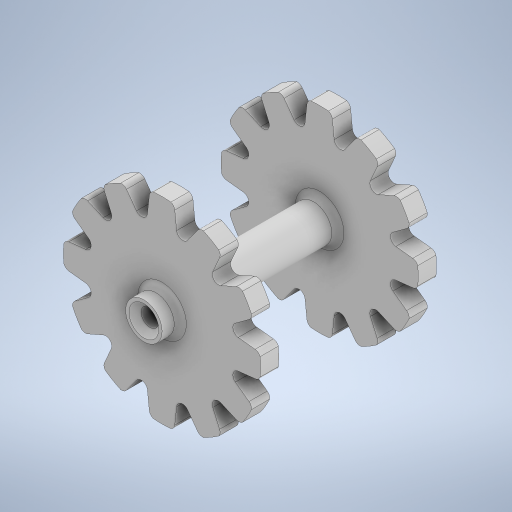
# Autodesk Inventor part: zebatka v12
Saved by Autodesk Inventor 2024 (Build 280153000, 153)
## iProperties
Created: 2025-03-28
Part Number: zebatka v12
Material: Ogólny
Document SubType Name: Modeling
Designer: Victoria
Density: 1 g/cm^3
Appearance: Domyślna
Author: Victoria
Autodesk Inventor part; units mm, degrees
ref_plane "YZ Plane" through (0, 0, 0) normal (1, 0, 0) x (0, 1, 0)
ref_plane "XZ Plane" through (0, 0, 0) normal (0, 1, 0) x (-1, 0, 0)
ref_plane "XY Plane" through (0, 0, 0) normal (0, 0, 1) x (1, 0, 0)
sketch "Szkic1" plane through (0, 0, 0) normal (0, 0, 1) x (1, 0, 0)
  circle A0 centre (0, 0) radius 16.25
  line L0 (0, 16.25) -> (-1.105, 16.25)
  line L1 (0, 16.25) -> (1.105, 16.25)
  line L2 (2.5, 11.75) -> (2.0988, 15.3604)
  line L3 (-2.5, 11.75) -> (-2.0988, 15.3604)
  arc A1 (-1.105, 16.25) -> (-2.0988, 15.3604) centre (-1.105, 15.25) ccw
  arc A2 (2.0988, 15.3604) -> (1.105, 16.25) centre (1.105, 15.25) ccw
  line L4 (3.7099, 11.4258) -> (5.8626, 14.3519)
  arc A3 (7.1681, 14.6254) -> (5.8626, 14.3519) centre (6.6681, 13.7594) ccw
  line L5 (8.125, 14.0729) -> (7.1681, 14.6254)
  line L6 (8.125, 14.0729) -> (9.0819, 13.5204)
  arc A4 (9.4979, 12.2531) -> (9.0819, 13.5204) centre (8.5819, 12.6544) ccw
  line L7 (8.0401, 8.9258) -> (9.4979, 12.2531)
  line L8 (8.9258, 8.0401) -> (12.2531, 9.4979)
  arc A5 (13.5204, 9.0819) -> (12.2531, 9.4979) centre (12.6544, 8.5819) ccw
  line L9 (14.0729, 8.125) -> (13.5204, 9.0819)
  line L10 (14.0729, 8.125) -> (14.6254, 7.1681)
  arc A6 (14.3519, 5.8626) -> (14.6254, 7.1681) centre (13.7594, 6.6681) ccw
  line L11 (11.4258, 3.7099) -> (14.3519, 5.8626)
  line L12 (11.75, 2.5) -> (15.3604, 2.0988)
  arc A7 (16.25, 1.105) -> (15.3604, 2.0988) centre (15.25, 1.105) ccw
  line L13 (16.25, 0) -> (16.25, 1.105)
  line L14 (16.25, 0) -> (16.25, -1.105)
  arc A8 (15.3604, -2.0988) -> (16.25, -1.105) centre (15.25, -1.105) ccw
  line L15 (11.75, -2.5) -> (15.3604, -2.0988)
  line L16 (11.4258, -3.7099) -> (14.3519, -5.8626)
  arc A9 (14.6254, -7.1681) -> (14.3519, -5.8626) centre (13.7594, -6.6681) ccw
  line L17 (14.0729, -8.125) -> (14.6254, -7.1681)
  line L18 (14.0729, -8.125) -> (13.5204, -9.0819)
  arc A10 (12.2531, -9.4979) -> (13.5204, -9.0819) centre (12.6544, -8.5819) ccw
  line L19 (8.9258, -8.0401) -> (12.2531, -9.4979)
  line L20 (8.0401, -8.9258) -> (9.4979, -12.2531)
  arc A11 (9.0819, -13.5204) -> (9.4979, -12.2531) centre (8.5819, -12.6544) ccw
  line L21 (8.125, -14.0729) -> (9.0819, -13.5204)
  line L22 (8.125, -14.0729) -> (7.1681, -14.6254)
  arc A12 (5.8626, -14.3519) -> (7.1681, -14.6254) centre (6.6681, -13.7594) ccw
  line L23 (3.7099, -11.4258) -> (5.8626, -14.3519)
  line L24 (2.5, -11.75) -> (2.0988, -15.3604)
  arc A13 (1.105, -16.25) -> (2.0988, -15.3604) centre (1.105, -15.25) ccw
  line L25 (0, -16.25) -> (1.105, -16.25)
  line L26 (0, -16.25) -> (-1.105, -16.25)
  arc A14 (-2.0988, -15.3604) -> (-1.105, -16.25) centre (-1.105, -15.25) ccw
  line L27 (-2.5, -11.75) -> (-2.0988, -15.3604)
  line L28 (-3.7099, -11.4258) -> (-5.8626, -14.3519)
  arc A15 (-7.1681, -14.6254) -> (-5.8626, -14.3519) centre (-6.6681, -13.7594) ccw
  line L29 (-8.125, -14.0729) -> (-7.1681, -14.6254)
  line L30 (-8.125, -14.0729) -> (-9.0819, -13.5204)
  arc A16 (-9.4979, -12.2531) -> (-9.0819, -13.5204) centre (-8.5819, -12.6544) ccw
  line L31 (-8.0401, -8.9258) -> (-9.4979, -12.2531)
  line L32 (-8.9258, -8.0401) -> (-12.2531, -9.4979)
  arc A17 (-13.5204, -9.0819) -> (-12.2531, -9.4979) centre (-12.6544, -8.5819) ccw
  line L33 (-14.0729, -8.125) -> (-13.5204, -9.0819)
  line L34 (-14.0729, -8.125) -> (-14.6254, -7.1681)
  arc A18 (-14.3519, -5.8626) -> (-14.6254, -7.1681) centre (-13.7594, -6.6681) ccw
  line L35 (-11.4258, -3.7099) -> (-14.3519, -5.8626)
  line L36 (-11.75, -2.5) -> (-15.3604, -2.0988)
  arc A19 (-16.25, -1.105) -> (-15.3604, -2.0988) centre (-15.25, -1.105) ccw
  line L37 (-16.25, 0) -> (-16.25, -1.105)
  line L38 (-16.25, 0) -> (-16.25, 1.105)
  arc A20 (-15.3604, 2.0988) -> (-16.25, 1.105) centre (-15.25, 1.105) ccw
  line L39 (-11.75, 2.5) -> (-15.3604, 2.0988)
  line L40 (-11.4258, 3.7099) -> (-14.3519, 5.8626)
  arc A21 (-14.6254, 7.1681) -> (-14.3519, 5.8626) centre (-13.7594, 6.6681) ccw
  line L41 (-14.0729, 8.125) -> (-14.6254, 7.1681)
  line L42 (-14.0729, 8.125) -> (-13.5204, 9.0819)
  arc A22 (-12.2531, 9.4979) -> (-13.5204, 9.0819) centre (-12.6544, 8.5819) ccw
  line L43 (-8.9258, 8.0401) -> (-12.2531, 9.4979)
  line L44 (-8.0401, 8.9258) -> (-9.4979, 12.2531)
  arc A23 (-9.0819, 13.5204) -> (-9.4979, 12.2531) centre (-8.5819, 12.6544) ccw
  line L45 (-8.125, 14.0729) -> (-9.0819, 13.5204)
  line L46 (-8.125, 14.0729) -> (-7.1681, 14.6254)
  arc A24 (-5.8626, 14.3519) -> (-7.1681, 14.6254) centre (-6.6681, 13.7594) ccw
  line L47 (-3.7099, 11.4258) -> (-5.8626, 14.3519)
  circle A25 centre (0, 0) radius 12.013
  circle A26 centre (0, 0) radius 1.45
  point P0 (-2, 16.25)
  point P1 (2, 16.25)
  point P2 (6.3929, 15.0729)
  point P3 (9.8571, 13.0729)
  point P4 (13.0729, 9.8571)
  point P5 (15.0729, 6.3929)
  point P6 (16.25, 2)
  point P7 (16.25, -2)
  point P8 (15.0729, -6.3929)
  point P9 (13.0729, -9.8571)
  point P10 (9.8571, -13.0729)
  point P11 (6.3929, -15.0729)
  point P12 (2, -16.25)
  point P13 (-2, -16.25)
  point P14 (-6.3929, -15.0729)
  point P15 (-9.8571, -13.0729)
  point P16 (-13.0729, -9.8571)
  point P17 (-15.0729, -6.3929)
  point P18 (-16.25, -2)
  point P19 (-16.25, 2)
  point P20 (-15.0729, 6.3929)
  point P21 (-13.0729, 9.8571)
  point P22 (-9.8571, 13.0729)
  point P23 (-6.3929, 15.0729)
  point P24 (14.7468, 6.826)
  point P25 (13.2849, 9.3581)
  point P26 (9.3581, 13.2849)
  point P27 (6.826, 14.7468)
  point P28 (1.462, 16.1841)
  point P29 (-1.462, 16.1841)
  point P30 (-6.826, 14.7468)
  point P31 (-9.3581, 13.2849)
  point P32 (-13.2849, 9.3581)
  point P33 (-14.7468, 6.826)
  point P34 (-16.1841, 1.462)
  point P35 (-16.1841, -1.462)
  point P36 (-14.7468, -6.826)
  point P37 (-13.2849, -9.3581)
  point P38 (-9.3581, -13.2849)
  point P39 (-6.826, -14.7468)
  point P40 (-1.462, -16.1841)
  point P41 (1.462, -16.1841)
  point P42 (6.826, -14.7468)
  point P43 (9.3581, -13.2849)
  point P44 (13.2849, -9.3581)
  point P45 (14.7468, -6.826)
  point P46 (16.1841, -1.462)
  point P47 (16.1841, 1.462)
  dimension "d0" = 32.5
  dimension "d2" = 2
  dimension "d3" = 2
  dimension "d6" = 1
  dimension "d9" = 360
  dimension "d11" = 2.9
  constraints: 96 end point, 60 point on line, 48 point on circle, 25 centre point, 4 coincident, 4 tangent, 2 horizontal, 1 equal radius, 221 other
  measures "d2" distance of L0.start point (-2, 16.25)
  measures "d3" distance of L0.start point (2, 16.25)
  measures "d6" radius of A1
  measures "d11" diameter of A26
extrude "Wyciągnięcie proste1" add sketch "Szkic1" along normal blind 3 contours A0 A8 L15 A25 L12 A7 | A6 L11 A25 L8 A5 A0 | A0 A10 L19 A25 L16 A9 | A25 | A4 L7 A25 L4 A3 A0 | A0 A12 L23 A25 L20 A11 | A2 L2 A25 L3 A1 A0 | A0 A14 L27 A25 L24 A13 | A25 L44 A23 A0 A24 L47 | L28 A15 A0 A16 L31 A25 | A25 L40 A21 A0 A22 L43 | L32 A17 A0 A18 L35 A25 | A25 L36 A19 A0 A20 L39
sketch "Szkic2" plane through (0, 0, 3) normal (0, 0, 1) x (1, 0, 0)
  circle A0 centre (0, 0) radius 3
  line L0 (11.4258, 3.7099) -> (14.3519, 5.8626) projected
  arc A1 (14.3519, 5.8626) -> (14.7468, 6.826) centre (13.7594, 6.6681) ccw projected
  arc A2 (14.7468, 6.826) -> (13.2849, 9.3581) centre (0, 0) ccw projected
  arc A3 (13.2849, 9.3581) -> (12.2531, 9.4979) centre (12.6544, 8.5819) ccw projected
  line L1 (12.2531, 9.4979) -> (8.9258, 8.0401) projected
  arc A4 (8.9258, 8.0401) -> (8.0401, 8.9258) centre (0, 0) ccw projected
  line L2 (8.0401, 8.9258) -> (9.4979, 12.2531) projected
  arc A5 (9.4979, 12.2531) -> (9.3581, 13.2849) centre (8.5819, 12.6544) ccw projected
  arc A6 (9.3581, 13.2849) -> (6.826, 14.7468) centre (0, 0) ccw projected
  arc A7 (6.826, 14.7468) -> (5.8626, 14.3519) centre (6.6681, 13.7594) ccw projected
  line L3 (5.8626, 14.3519) -> (3.7099, 11.4258) projected
  arc A8 (3.7099, 11.4258) -> (2.5, 11.75) centre (0, 0) ccw projected
  line L4 (2.5, 11.75) -> (2.0988, 15.3604) projected
  arc A9 (2.0988, 15.3604) -> (1.462, 16.1841) centre (1.105, 15.25) ccw projected
  arc A10 (1.462, 16.1841) -> (-1.462, 16.1841) centre (0, 0) ccw projected
  arc A11 (-1.462, 16.1841) -> (-2.0988, 15.3604) centre (-1.105, 15.25) ccw projected
  line L5 (-2.0988, 15.3604) -> (-2.5, 11.75) projected
  arc A12 (-2.5, 11.75) -> (-3.7099, 11.4258) centre (0, 0) ccw projected
  line L6 (-3.7099, 11.4258) -> (-5.8626, 14.3519) projected
  arc A13 (-5.8626, 14.3519) -> (-6.826, 14.7468) centre (-6.6681, 13.7594) ccw projected
  arc A14 (-6.826, 14.7468) -> (-9.3581, 13.2849) centre (0, 0) ccw projected
  arc A15 (-9.3581, 13.2849) -> (-9.4979, 12.2531) centre (-8.5819, 12.6544) ccw projected
  line L7 (-9.4979, 12.2531) -> (-8.0401, 8.9258) projected
  arc A16 (-8.0401, 8.9258) -> (-8.9258, 8.0401) centre (0, 0) ccw projected
  line L8 (-8.9258, 8.0401) -> (-12.2531, 9.4979) projected
  arc A17 (-12.2531, 9.4979) -> (-13.2849, 9.3581) centre (-12.6544, 8.5819) ccw projected
  arc A18 (-13.2849, 9.3581) -> (-14.7468, 6.826) centre (0, 0) ccw projected
  arc A19 (-14.7468, 6.826) -> (-14.3519, 5.8626) centre (-13.7594, 6.6681) ccw projected
  line L9 (-14.3519, 5.8626) -> (-11.4258, 3.7099) projected
  arc A20 (-11.4258, 3.7099) -> (-11.75, 2.5) centre (0, 0) ccw projected
  line L10 (-11.75, 2.5) -> (-15.3604, 2.0988) projected
  arc A21 (-15.3604, 2.0988) -> (-16.1841, 1.462) centre (-15.25, 1.105) ccw projected
  arc A22 (-16.1841, 1.462) -> (-16.1841, -1.462) centre (0, 0) ccw projected
  arc A23 (-16.1841, -1.462) -> (-15.3604, -2.0988) centre (-15.25, -1.105) ccw projected
  line L11 (-15.3604, -2.0988) -> (-11.75, -2.5) projected
  arc A24 (-11.75, -2.5) -> (-11.4258, -3.7099) centre (0, 0) ccw projected
  line L12 (-11.4258, -3.7099) -> (-14.3519, -5.8626) projected
  arc A25 (-14.3519, -5.8626) -> (-14.7468, -6.826) centre (-13.7594, -6.6681) ccw projected
  arc A26 (-14.7468, -6.826) -> (-13.2849, -9.3581) centre (0, 0) ccw projected
  arc A27 (-13.2849, -9.3581) -> (-12.2531, -9.4979) centre (-12.6544, -8.5819) ccw projected
  line L13 (-12.2531, -9.4979) -> (-8.9258, -8.0401) projected
  arc A28 (-8.9258, -8.0401) -> (-8.0401, -8.9258) centre (0, 0) ccw projected
  line L14 (-8.0401, -8.9258) -> (-9.4979, -12.2531) projected
  arc A29 (-9.4979, -12.2531) -> (-9.3581, -13.2849) centre (-8.5819, -12.6544) ccw projected
  arc A30 (-9.3581, -13.2849) -> (-6.826, -14.7468) centre (0, 0) ccw projected
  arc A31 (-6.826, -14.7468) -> (-5.8626, -14.3519) centre (-6.6681, -13.7594) ccw projected
  line L15 (-5.8626, -14.3519) -> (-3.7099, -11.4258) projected
  arc A32 (-3.7099, -11.4258) -> (-2.5, -11.75) centre (0, 0) ccw projected
  line L16 (-2.5, -11.75) -> (-2.0988, -15.3604) projected
  arc A33 (-2.0988, -15.3604) -> (-1.462, -16.1841) centre (-1.105, -15.25) ccw projected
  arc A34 (-1.462, -16.1841) -> (1.462, -16.1841) centre (0, 0) ccw projected
  arc A35 (1.462, -16.1841) -> (2.0988, -15.3604) centre (1.105, -15.25) ccw projected
  line L17 (2.0988, -15.3604) -> (2.5, -11.75) projected
  arc A36 (2.5, -11.75) -> (3.7099, -11.4258) centre (0, 0) ccw projected
  line L18 (3.7099, -11.4258) -> (5.8626, -14.3519) projected
  arc A37 (5.8626, -14.3519) -> (6.826, -14.7468) centre (6.6681, -13.7594) ccw projected
  arc A38 (6.826, -14.7468) -> (9.3581, -13.2849) centre (0, 0) ccw projected
  arc A39 (9.3581, -13.2849) -> (9.4979, -12.2531) centre (8.5819, -12.6544) ccw projected
  line L19 (9.4979, -12.2531) -> (8.0401, -8.9258) projected
  arc A40 (8.0401, -8.9258) -> (8.9258, -8.0401) centre (0, 0) ccw projected
  line L20 (8.9258, -8.0401) -> (12.2531, -9.4979) projected
  arc A41 (12.2531, -9.4979) -> (13.2849, -9.3581) centre (12.6544, -8.5819) ccw projected
  arc A42 (13.2849, -9.3581) -> (14.7468, -6.826) centre (0, 0) ccw projected
  arc A43 (14.7468, -6.826) -> (14.3519, -5.8626) centre (13.7594, -6.6681) ccw projected
  line L21 (14.3519, -5.8626) -> (11.4258, -3.7099) projected
  arc A44 (11.4258, -3.7099) -> (11.75, -2.5) centre (0, 0) ccw projected
  line L22 (11.75, -2.5) -> (15.3604, -2.0988) projected
  arc A45 (15.3604, -2.0988) -> (16.1841, -1.462) centre (15.25, -1.105) ccw projected
  arc A46 (16.1841, -1.462) -> (16.1841, 1.462) centre (0, 0) ccw projected
  arc A47 (16.1841, 1.462) -> (15.3604, 2.0988) centre (15.25, 1.105) ccw projected
  line L23 (15.3604, 2.0988) -> (11.75, 2.5) projected
  arc A48 (11.75, 2.5) -> (11.4258, 3.7099) centre (0, 0) ccw projected
  circle A49 centre (0, 0) radius 1.45 projected
  dimension "d16" = 6
  constraints: 1 centre point, 1 coincident
  measures "d16" diameter of A0
extrude "Wyciągnięcie proste2" add sketch "Szkic2" along normal blind 3 and the other way blind 26 contours A0
sketch "Szkic3" plane through (0, 0, -23) normal (0, 0, -1) x (-1, 0, 0)
  circle A0 centre (0, 0) radius 3 projected
  line L0 (-11.4258, 3.7099) -> (-14.3519, 5.8626) projected
  arc A1 (-11.4258, 3.7099) -> (-11.75, 2.5) centre (0, 0) ccw projected
  line L1 (-15.3604, 2.0988) -> (-11.75, 2.5) projected
  arc A2 (-15.3604, 2.0988) -> (-16.1841, 1.462) centre (-15.25, 1.105) ccw projected
  arc A3 (-16.1841, 1.462) -> (-16.1841, -1.462) centre (0, 0) ccw projected
  arc A4 (-16.1841, -1.462) -> (-15.3604, -2.0988) centre (-15.25, -1.105) ccw projected
  line L2 (-11.75, -2.5) -> (-15.3604, -2.0988) projected
  arc A5 (-11.75, -2.5) -> (-11.4258, -3.7099) centre (0, 0) ccw projected
  line L3 (-14.3519, -5.8626) -> (-11.4258, -3.7099) projected
  arc A6 (-14.3519, -5.8626) -> (-14.7468, -6.826) centre (-13.7594, -6.6681) ccw projected
  arc A7 (-14.7468, -6.826) -> (-13.2849, -9.3581) centre (0, 0) ccw projected
  arc A8 (-13.2849, -9.3581) -> (-12.2531, -9.4979) centre (-12.6544, -8.5819) ccw projected
  line L4 (-8.9258, -8.0401) -> (-12.2531, -9.4979) projected
  arc A9 (-8.9258, -8.0401) -> (-8.0401, -8.9258) centre (0, 0) ccw projected
  line L5 (-9.4979, -12.2531) -> (-8.0401, -8.9258) projected
  arc A10 (-9.4979, -12.2531) -> (-9.3581, -13.2849) centre (-8.5819, -12.6544) ccw projected
  arc A11 (-9.3581, -13.2849) -> (-6.826, -14.7468) centre (0, 0) ccw projected
  arc A12 (-6.826, -14.7468) -> (-5.8626, -14.3519) centre (-6.6681, -13.7594) ccw projected
  line L6 (-3.7099, -11.4258) -> (-5.8626, -14.3519) projected
  arc A13 (-3.7099, -11.4258) -> (-2.5, -11.75) centre (0, 0) ccw projected
  line L7 (-2.0988, -15.3604) -> (-2.5, -11.75) projected
  arc A14 (-2.0988, -15.3604) -> (-1.462, -16.1841) centre (-1.105, -15.25) ccw projected
  arc A15 (-1.462, -16.1841) -> (1.462, -16.1841) centre (0, 0) ccw projected
  arc A16 (1.462, -16.1841) -> (2.0988, -15.3604) centre (1.105, -15.25) ccw projected
  line L8 (2.5, -11.75) -> (2.0988, -15.3604) projected
  arc A17 (2.5, -11.75) -> (3.7099, -11.4258) centre (0, 0) ccw projected
  line L9 (5.8626, -14.3519) -> (3.7099, -11.4258) projected
  arc A18 (5.8626, -14.3519) -> (6.826, -14.7468) centre (6.6681, -13.7594) ccw projected
  arc A19 (6.826, -14.7468) -> (9.3581, -13.2849) centre (0, 0) ccw projected
  arc A20 (9.3581, -13.2849) -> (9.4979, -12.2531) centre (8.5819, -12.6544) ccw projected
  line L10 (8.0401, -8.9258) -> (9.4979, -12.2531) projected
  arc A21 (8.0401, -8.9258) -> (8.9258, -8.0401) centre (0, 0) ccw projected
  line L11 (12.2531, -9.4979) -> (8.9258, -8.0401) projected
  arc A22 (12.2531, -9.4979) -> (13.2849, -9.3581) centre (12.6544, -8.5819) ccw projected
  arc A23 (13.2849, -9.3581) -> (14.7468, -6.826) centre (0, 0) ccw projected
  arc A24 (14.7468, -6.826) -> (14.3519, -5.8626) centre (13.7594, -6.6681) ccw projected
  line L12 (11.4258, -3.7099) -> (14.3519, -5.8626) projected
  arc A25 (11.4258, -3.7099) -> (11.75, -2.5) centre (0, 0) ccw projected
  line L13 (15.3604, -2.0988) -> (11.75, -2.5) projected
  arc A26 (15.3604, -2.0988) -> (16.1841, -1.462) centre (15.25, -1.105) ccw projected
  arc A27 (16.1841, -1.462) -> (16.1841, 1.462) centre (0, 0) ccw projected
  arc A28 (16.1841, 1.462) -> (15.3604, 2.0988) centre (15.25, 1.105) ccw projected
  line L14 (11.75, 2.5) -> (15.3604, 2.0988) projected
  arc A29 (11.75, 2.5) -> (11.4258, 3.7099) centre (0, 0) ccw projected
  line L15 (14.3519, 5.8626) -> (11.4258, 3.7099) projected
  arc A30 (14.3519, 5.8626) -> (14.7468, 6.826) centre (13.7594, 6.6681) ccw projected
  arc A31 (14.7468, 6.826) -> (13.2849, 9.3581) centre (0, 0) ccw projected
  arc A32 (13.2849, 9.3581) -> (12.2531, 9.4979) centre (12.6544, 8.5819) ccw projected
  line L16 (8.9258, 8.0401) -> (12.2531, 9.4979) projected
  arc A33 (8.9258, 8.0401) -> (8.0401, 8.9258) centre (0, 0) ccw projected
  line L17 (9.4979, 12.2531) -> (8.0401, 8.9258) projected
  arc A34 (9.4979, 12.2531) -> (9.3581, 13.2849) centre (8.5819, 12.6544) ccw projected
  arc A35 (9.3581, 13.2849) -> (6.826, 14.7468) centre (0, 0) ccw projected
  arc A36 (6.826, 14.7468) -> (5.8626, 14.3519) centre (6.6681, 13.7594) ccw projected
  line L18 (3.7099, 11.4258) -> (5.8626, 14.3519) projected
  arc A37 (3.7099, 11.4258) -> (2.5, 11.75) centre (0, 0) ccw projected
  line L19 (2.0988, 15.3604) -> (2.5, 11.75) projected
  arc A38 (2.0988, 15.3604) -> (1.462, 16.1841) centre (1.105, 15.25) ccw projected
  arc A39 (1.462, 16.1841) -> (-1.462, 16.1841) centre (0, 0) ccw projected
  arc A40 (-1.462, 16.1841) -> (-2.0988, 15.3604) centre (-1.105, 15.25) ccw projected
  line L20 (-2.5, 11.75) -> (-2.0988, 15.3604) projected
  arc A41 (-2.5, 11.75) -> (-3.7099, 11.4258) centre (0, 0) ccw projected
  line L21 (-5.8626, 14.3519) -> (-3.7099, 11.4258) projected
  arc A42 (-5.8626, 14.3519) -> (-6.826, 14.7468) centre (-6.6681, 13.7594) ccw projected
  arc A43 (-6.826, 14.7468) -> (-9.3581, 13.2849) centre (0, 0) ccw projected
  arc A44 (-9.3581, 13.2849) -> (-9.4979, 12.2531) centre (-8.5819, 12.6544) ccw projected
  line L22 (-8.0401, 8.9258) -> (-9.4979, 12.2531) projected
  arc A45 (-8.0401, 8.9258) -> (-8.9258, 8.0401) centre (0, 0) ccw projected
  line L23 (-12.2531, 9.4979) -> (-8.9258, 8.0401) projected
  arc A46 (-12.2531, 9.4979) -> (-13.2849, 9.3581) centre (-12.6544, 8.5819) ccw projected
  arc A47 (-13.2849, 9.3581) -> (-14.7468, 6.826) centre (0, 0) ccw projected
  arc A48 (-14.7468, 6.826) -> (-14.3519, 5.8626) centre (-13.7594, 6.6681) ccw projected
  circle A49 centre (0, 0) radius 3 projected
  circle A50 centre (0, 0) radius 1.45 projected
extrude "Wyciągnięcie proste3" add sketch "Szkic3" along normal blind 3 contours A0 | L0 A48 A47 A46 L23 A45 L22 A44 A43 A42 L21 A41 L20 A40 A39 A38 L19 A37 L18 A36 A35 A34 L17 A33 L16 A32 A31 A30 L15 A29 L14 A28 A27 A26 L13 A25 L12 A24 A23 A22 L11 A21 L10 A20 A19 A18 L9 A17 L8 A16 A15 A14 L7 A13 L6 A12 A11 A10 L5 A9 L4 A8 A7 A6 L3 A5 L2 A4 A3 A2 L1 A1
sketch "Szkic4" plane through (0, 0, -26) normal (0, 0, -1) x (-1, 0, 0)
  circle A0 centre (0, 0) radius 3 projected
  circle A1 centre (0, 0) radius 3 projected
  circle A2 centre (0, 0) radius 1.45 projected
  circle A3 centre (0, 0) radius 1.45 projected
extrude "Wyciągnięcie proste4" add sketch "Szkic4" along normal blind 5
fillet "Zaokrąglenie1" radius 1 4 edges at (3, 0, -26) (-3, 0, -23) (-3, 0, 0) (-3, 0, 3)
chamfer "Faza1" distance 1 angle 45 2 edges at (1.45, 0, -31) (-1.45, 0, 6)
fillet "Zaokrąglenie2" radius 1 48 edges at (11.75, 2.5, -24.5) (11.4258, 3.7099, -24.5) (8.9258, 8.0401, -24.5) (8.0401, 8.9258, -24.5) (3.7099, 11.4258, -24.5) (2.5, 11.75, -24.5) (-2.5, 11.75, -24.5) (-3.7099, 11.4258, -24.5) (-8.0401, 8.9258, -24.5) (-11.4258, 3.7099, -24.5) (-11.75, 2.5, -24.5) (-8.9258, 8.0401, -24.5) (-2.5, 11.75, 1.5) (-3.7099, 11.4258, 1.5) (3.7099, 11.4258, 1.5) (2.5, 11.75, 1.5) (8.0401, 8.9258, 1.5) (8.9258, 8.0401, 1.5) (11.4258, 3.7099, 1.5) (11.75, 2.5, 1.5) (-8.0401, 8.9258, 1.5) (-8.9258, 8.0401, 1.5) (-11.75, 2.5, 1.5) (-11.4258, 3.7099, 1.5) (-11.75, -2.5, 1.5) (-11.4258, -3.7099, 1.5) (-8.9258, -8.0401, 1.5) (-8.0401, -8.9258, 1.5) (-3.7099, -11.4258, 1.5) (-2.5, -11.75, 1.5) (2.5, -11.75, 1.5) (3.7099, -11.4258, 1.5) (8.0401, -8.9258, 1.5) (8.9258, -8.0401, 1.5) (-11.75, -2.5, -24.5) (-11.4258, -3.7099, -24.5) (-8.9258, -8.0401, -24.5) (-8.0401, -8.9258, -24.5) (-3.7099, -11.4258, -24.5) (-2.5, -11.75, -24.5) (2.5, -11.75, -24.5) (3.7099, -11.4258, -24.5) (8.0401, -8.9258, -24.5) (8.9258, -8.0401, -24.5) (11.4258, -3.7099, -24.5) (11.75, -2.5, -24.5) (11.4258, -3.7099, 1.5) (11.75, -2.5, 1.5)
